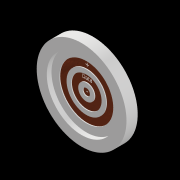
# Autodesk Inventor part: Connector
Saved by Autodesk Inventor 2022.1 (Build 261234000, 234)
## iProperties
Created: 2022-01-31
Part Number: Connector
Material: Generic
Document SubType Name: Modeling
Designer: Michael Lacey
Mass: 1.54155 g
Surface Area: 15.3616 cm^2
Volume: 1.54155 cm^3
Density: 1 g/cm^3
Appearance: Default
Author: Michael Lacey
Autodesk Inventor part; units mm, degrees
ref_plane "YZ Plane" through (0, 0, 0) normal (1, 0, 0) x (0, 1, 0)
ref_plane "XZ Plane" through (0, 0, 0) normal (0, 1, 0) x (-1, 0, 0)
ref_plane "XY Plane" through (0, 0, 0) normal (0, 0, 1) x (1, 0, 0)
sketch "Sketch1" plane through (0, 0, 0) normal (0, 0, 1) x (1, 0, 0)
  circle A0 centre (0, 0) radius 12.7 projected
  circle A1 centre (0, 0) radius 11.1125 construction
  circle A2 centre (0, 0) radius 9.8425
  dimension "d0" = 1.27
  constraints: 1 centre point, 1 coincident
  measures "d0" radial gap between concentric circles of A1 A2
extrude "Extrusion1" add sketch "Sketch1" along normal blind 3.175
sketch "Sketch2" plane through (0, 0, 0) normal (0, 0, -1) x (-1, 0, 0)
  circle A0 centre (0, 0) radius 1.016
  circle A1 centre (0, 0) radius 2.286
  circle A2 centre (0, 0) radius 4.318
  circle A3 centre (0, 0) radius 5.588
  circle A4 centre (0, 0) radius 7.62
  dimension "d3" = 2.032
  dimension "d4" = 2.032
  dimension "d5" = 2.032
  dimension "d6" = 1.27
  dimension "d7" = 1.27
  constraints: 5 centre point, 5 coincident
  measures "d3" diameter of A0
  measures "d4" radial gap between concentric circles of A2 A1
  measures "d5" radial gap between concentric circles of A4 A3
  measures "d6" radial gap between concentric circles of A1 A0
  measures "d7" radial gap between concentric circles of A3 A2
extrude "Extrusion2" add sketch "Sketch2" along normal mid plane 3.175
sketch "Sketch3" plane through (0, 0, 1.5875) normal (0, 0, 1) x (1, 0, 0)
  line L0 (-0.635, 7.239) -> (0.635, 7.239) construction
  line L1 (0.635, 7.239) -> (0.635, 5.969) construction
  line L2 (0.635, 5.969) -> (-0.635, 5.969) construction
  line L3 (-0.635, 5.969) -> (-0.635, 7.239) construction
  circle A0 centre (0, 0) radius 7.62 projected
  circle A1 centre (0, 0) radius 5.588 projected
  circle A2 centre (0, 0) radius 4.318 projected
  circle A3 centre (0, 0) radius 2.286 projected
  circle A4 centre (0, 0) radius 1.016 projected
  line L4 (0, 5.588) -> (0, 5.969) construction
  line L5 (0, 7.239) -> (0, 7.62) construction
  line L6 (-0.2762, 0.2762) -> (0.2762, 0.2762) construction
  line L7 (0.2762, 0.2762) -> (0.2762, -0.2762) construction
  line L8 (0.2762, -0.2762) -> (-0.2762, -0.2762) construction
  line L9 (-0.2762, -0.2762) -> (-0.2762, 0.2762) construction
  line L10 (0, 0.2762) -> (0, 1.016) construction
  line L11 (0.2762, 0) -> (1.016, 0) construction
  line L12 (0, -0.2762) -> (0, -1.016) construction
  line L13 (-0.2762, 0) -> (-1.016, 0) construction
  line L14 (-1.016, 4.318) -> (1.016, 4.318) construction
  line L15 (1.016, 4.318) -> (1.016, 2.286) construction
  line L16 (1.016, 2.286) -> (-1.016, 2.286) construction
  line L17 (-1.016, 2.286) -> (-1.016, 4.318) construction
  line L18 (0.5017, 6.5356) -> (0.0715, 6.5356)
  line L19 (0.0715, 6.5356) -> (0.0715, 6.1054)
  line L20 (0.0715, 6.1054) -> (-0.0705, 6.1054)
  line L21 (-0.0705, 6.1054) -> (-0.0705, 6.5356)
  line L22 (-0.0705, 6.5356) -> (-0.5007, 6.5356)
  line L23 (-0.5007, 6.5356) -> (-0.5007, 6.6724)
  line L24 (-0.5007, 6.6724) -> (-0.0705, 6.6724)
  line L25 (-0.0705, 6.6724) -> (-0.0705, 7.1026)
  line L26 (-0.0705, 7.1026) -> (0.0715, 7.1026)
  line L27 (0.0715, 7.1026) -> (0.0715, 6.6724)
  line L28 (0.0715, 6.6724) -> (0.5017, 6.6724)
  line L29 (0.5017, 6.6724) -> (0.5017, 6.5356)
  spline S0 degree 2 poles (-0.5372, 3.3119) (-0.5372, 3.1727) (-0.65, 2.9488) (-0.7447, 2.8862) knots 0 0 0 1 2 2 2
  spline S1 degree 2 poles (-0.7447, 2.8862) (-0.8221, 2.8376) (-0.981, 2.8047) (-1.1045, 2.8047) knots 0 0 0 1 2 2 2
  line L30 (-1.1045, 2.8047) -> (-1.3383, 2.8047)
  line L31 (-1.3383, 2.8047) -> (-1.3383, 3.8207)
  line L32 (-1.3383, 3.8207) -> (-1.107, 3.8207)
  spline S2 degree 2 poles (-1.107, 3.8207) (-0.9637, 3.8207) (-0.8007, 3.7779) (-0.7431, 3.74) knots 0 0 0 1 2 2 2
  spline S3 degree 2 poles (-0.7431, 3.74) (-0.6451, 3.675) (-0.5372, 3.4601) (-0.5372, 3.3119) knots 0 0 0 1 2 2 2
  spline S4 degree 2 poles (-0.678, 3.3135) (-0.678, 3.4304) (-0.7554, 3.5959) (-0.832, 3.6429) knots 0 0 0 1 2 2 2
  spline S5 degree 2 poles (-0.832, 3.6429) (-0.8863, 3.675) (-1.009, 3.7038) (-1.1004, 3.7038) knots 0 0 0 1 2 2 2
  line L33 (-1.1004, 3.7038) -> (-1.2033, 3.7038)
  line L34 (-1.2033, 3.7038) -> (-1.2033, 2.9216)
  line L35 (-1.2033, 2.9216) -> (-1.1004, 2.9216)
  spline S6 degree 2 poles (-1.1004, 2.9216) (-1.0106, 2.9216) (-0.8748, 2.9504) (-0.8196, 2.9891) knots 0 0 0 1 2 2 2
  spline S7 degree 2 poles (-0.8196, 2.9891) (-0.7488, 3.0369) (-0.678, 3.195) (-0.678, 3.3135) knots 0 0 0 1 2 2 2
  spline S8 degree 2 poles (0.0243, 2.8854) (0.0086, 2.8739) (-0.044, 2.8327) (-0.0687, 2.8203) knots 0 0 0 1 2 2 2
  spline S9 degree 2 poles (-0.0687, 2.8203) (-0.1025, 2.8022) (-0.1659, 2.7833) (-0.2235, 2.7833) knots 0 0 0 1 2 2 2
  spline S10 degree 2 poles (-0.2235, 2.7833) (-0.2705, 2.7833) (-0.3553, 2.8187) (-0.3874, 2.8508) knots 0 0 0 1 2 2 2
  spline S11 degree 2 poles (-0.3874, 2.8508) (-0.4178, 2.8821) (-0.4549, 2.9743) (-0.4549, 3.0254) knots 0 0 0 1 2 2 2
  spline S12 degree 2 poles (-0.4549, 3.0254) (-0.4549, 3.1044) (-0.3882, 3.2164) (-0.3158, 3.2485) knots 0 0 0 1 2 2 2
  spline S13 degree 2 poles (-0.3158, 3.2485) (-0.2515, 3.2781) (-0.077, 3.3004) (0.0243, 3.3061) knots 0 0 0 1 2 2 2
  line L36 (0.0243, 3.3061) -> (0.0243, 3.3308)
  spline S14 degree 2 poles (0.0243, 3.3308) (0.0243, 3.3753) (-0.0029, 3.4304) (-0.0276, 3.4461) knots 0 0 0 1 2 2 2
  spline S15 degree 2 poles (-0.0276, 3.4461) (-0.0523, 3.4617) (-0.1231, 3.4716) (-0.161, 3.4716) knots 0 0 0 1 2 2 2
  spline S16 degree 2 poles (-0.161, 3.4716) (-0.2054, 3.4716) (-0.3256, 3.4453) (-0.3857, 3.4197) knots 0 0 0 1 2 2 2
  line L37 (-0.3857, 3.4197) -> (-0.3931, 3.4197)
  line L38 (-0.3931, 3.4197) -> (-0.3931, 3.5506)
  spline S17 degree 2 poles (-0.3931, 3.5506) (-0.3577, 3.5605) (-0.2252, 3.5852) (-0.1601, 3.5852) knots 0 0 0 1 2 2 2
  spline S18 degree 2 poles (-0.1601, 3.5852) (-0.0811, 3.5852) (0.0268, 3.5605) (0.0696, 3.5284) knots 0 0 0 1 2 2 2
  spline S19 degree 2 poles (0.0696, 3.5284) (0.1116, 3.4971) (0.1527, 3.3975) (0.1527, 3.3259) knots 0 0 0 1 2 2 2
  line L39 (0.1527, 3.3259) -> (0.1527, 2.8047)
  line L40 (0.1527, 2.8047) -> (0.0243, 2.8047)
  line L41 (0.0243, 2.8047) -> (0.0243, 2.8854)
  line L42 (0.0243, 2.9924) -> (0.0243, 3.204)
  spline S20 degree 2 poles (0.0243, 3.204) (-0.0218, 3.1999) (-0.161, 3.1859) (-0.2046, 3.1727) knots 0 0 0 1 2 2 2
  spline S21 degree 2 poles (-0.2046, 3.1727) (-0.2556, 3.1571) (-0.3223, 3.092) (-0.3223, 3.0344) knots 0 0 0 1 2 2 2
  spline S22 degree 2 poles (-0.3223, 3.0344) (-0.3223, 2.9685) (-0.2482, 2.9019) (-0.1774, 2.9019) knots 0 0 0 1 2 2 2
  spline S23 degree 2 poles (-0.1774, 2.9019) (-0.1173, 2.9019) (-0.0185, 2.9537) (0.0243, 2.9924) knots 0 0 0 1 2 2 2
  spline S24 degree 2 poles (0.5636, 2.7899) (0.459, 2.7899) (0.3413, 2.9093) (0.3413, 3.0385) knots 0 0 0 1 2 2 2
  line L43 (0.3413, 3.0385) -> (0.3413, 3.4609)
  line L44 (0.3413, 3.4609) -> (0.2548, 3.4609)
  line L45 (0.2548, 3.4609) -> (0.2548, 3.5671)
  line L46 (0.2548, 3.5671) -> (0.3413, 3.5671)
  line L47 (0.3413, 3.5671) -> (0.3413, 3.7861)
  line L48 (0.3413, 3.7861) -> (0.4697, 3.7861)
  line L49 (0.4697, 3.7861) -> (0.4697, 3.5671)
  line L50 (0.4697, 3.5671) -> (0.706, 3.5671)
  line L51 (0.706, 3.5671) -> (0.706, 3.4609)
  line L52 (0.706, 3.4609) -> (0.4697, 3.4609)
  line L53 (0.4697, 3.4609) -> (0.4697, 3.0978)
  spline S25 degree 2 poles (0.4697, 3.0978) (0.4697, 3.0402) (0.4738, 2.9768) (0.4878, 2.9496) knots 0 0 0 1 2 2 2
  spline S26 degree 2 poles (0.4878, 2.9496) (0.4994, 2.9257) (0.5512, 2.9019) (0.5957, 2.9019) knots 0 0 0 1 2 2 2
  spline S27 degree 2 poles (0.5957, 2.9019) (0.627, 2.9019) (0.6854, 2.9208) (0.6986, 2.9266) knots 0 0 0 1 2 2 2
  line L54 (0.6986, 2.9266) -> (0.706, 2.9266)
  line L55 (0.706, 2.9266) -> (0.706, 2.8113)
  spline S28 degree 2 poles (0.706, 2.8113) (0.6698, 2.8014) (0.5957, 2.7899) (0.5636, 2.7899) knots 0 0 0 1 2 2 2
  spline S29 degree 2 poles (1.2255, 2.8854) (1.2099, 2.8739) (1.1572, 2.8327) (1.1325, 2.8203) knots 0 0 0 1 2 2 2
  spline S30 degree 2 poles (1.1325, 2.8203) (1.0987, 2.8022) (1.0353, 2.7833) (0.9777, 2.7833) knots 0 0 0 1 2 2 2
  spline S31 degree 2 poles (0.9777, 2.7833) (0.9308, 2.7833) (0.846, 2.8187) (0.8139, 2.8508) knots 0 0 0 1 2 2 2
  spline S32 degree 2 poles (0.8139, 2.8508) (0.7834, 2.8821) (0.7464, 2.9743) (0.7464, 3.0254) knots 0 0 0 1 2 2 2
  spline S33 degree 2 poles (0.7464, 3.0254) (0.7464, 3.1044) (0.813, 3.2164) (0.8855, 3.2485) knots 0 0 0 1 2 2 2
  spline S34 degree 2 poles (0.8855, 3.2485) (0.9497, 3.2781) (1.1243, 3.3004) (1.2255, 3.3061) knots 0 0 0 1 2 2 2
  line L56 (1.2255, 3.3061) -> (1.2255, 3.3308)
  spline S35 degree 2 poles (1.2255, 3.3308) (1.2255, 3.3753) (1.1984, 3.4304) (1.1737, 3.4461) knots 0 0 0 1 2 2 2
  spline S36 degree 2 poles (1.1737, 3.4461) (1.149, 3.4617) (1.0782, 3.4716) (1.0403, 3.4716) knots 0 0 0 1 2 2 2
  spline S37 degree 2 poles (1.0403, 3.4716) (0.9958, 3.4716) (0.8756, 3.4453) (0.8155, 3.4197) knots 0 0 0 1 2 2 2
  line L57 (0.8155, 3.4197) -> (0.8081, 3.4197)
  line L58 (0.8081, 3.4197) -> (0.8081, 3.5506)
  spline S38 degree 2 poles (0.8081, 3.5506) (0.8435, 3.5605) (0.9761, 3.5852) (1.0411, 3.5852) knots 0 0 0 1 2 2 2
  spline S39 degree 2 poles (1.0411, 3.5852) (1.1202, 3.5852) (1.228, 3.5605) (1.2708, 3.5284) knots 0 0 0 1 2 2 2
  spline S40 degree 2 poles (1.2708, 3.5284) (1.3128, 3.4971) (1.354, 3.3975) (1.354, 3.3259) knots 0 0 0 1 2 2 2
  line L59 (1.354, 3.3259) -> (1.354, 2.8047)
  line L60 (1.354, 2.8047) -> (1.2255, 2.8047)
  line L61 (1.2255, 2.8047) -> (1.2255, 2.8854)
  line L62 (1.2255, 2.9924) -> (1.2255, 3.204)
  spline S41 degree 2 poles (1.2255, 3.204) (1.1794, 3.1999) (1.0403, 3.1859) (0.9967, 3.1727) knots 0 0 0 1 2 2 2
  spline S42 degree 2 poles (0.9967, 3.1727) (0.9456, 3.1571) (0.8789, 3.092) (0.8789, 3.0344) knots 0 0 0 1 2 2 2
  spline S43 degree 2 poles (0.8789, 3.0344) (0.8789, 2.9685) (0.953, 2.9019) (1.0238, 2.9019) knots 0 0 0 1 2 2 2
  spline S44 degree 2 poles (1.0238, 2.9019) (1.0839, 2.9019) (1.1827, 2.9537) (1.2255, 2.9924) knots 0 0 0 1 2 2 2
  line L63 (0.2408, -0.0772) -> (-0.2398, -0.0772)
  line L64 (-0.2398, -0.0772) -> (-0.2398, 0.0772)
  line L65 (-0.2398, 0.0772) -> (0.2408, 0.0772)
  line L66 (0.2408, 0.0772) -> (0.2408, -0.0772)
  point P0 (0, 2.286)
  point P1 (0, 4.318)
  point P2 (2.886, -2.4456)
  point P3 (2.886, 0.3842)
  dimension "d12" = 1.27
  constraints: 12 end point, 8 midpoint, 6 equal length, 6 vertical alignment, 4 point on circle, 3 horizontal, 2 point on line, 2 vertical, 1 horizontal alignment, 10 other
  measures "d12" distance of L0.end L1.end
extrude "Extrusion3" cut sketch "Sketch3" against normal blind 0.508 contours L18 L19 L20 L21 L22 L23 L24 L25 L26 L27 L28 L29 | S0 S1 L30 L31 L32 S2 S3 | S8 S9 S10 S11 S12 S13 L36 S14 S15 S16 L37 L38 S17 S18 S19 L39 L40 L41 | S24 L43 L44 L45 L46 L47 L48 L49 L50 L51 L52 L53 S25 S26 S27 L54 L55 S28 | S29 S30 S31 S32 S33 S34 L56 S35 S36 S37 L57 L58 S38 S39 S40 L59 L60 L61 | L63 L64 L65 L66
sketch "Sketch4" plane through (0, 0, 1.5875) normal (0, 0, 1) x (1, 0, 0)
  circle A0 centre (0, 0) radius 2.286 projected
  circle A1 centre (0, 0) radius 4.318 projected
  line L0 (1.2255, 2.8047) -> (1.2255, 2.8854) projected
  line L1 (1.2255, 3.3061) -> (1.2255, 3.3308) projected
  line L2 (0.8155, 3.4197) -> (0.8081, 3.4197) projected
  line L3 (0.8081, 3.4197) -> (0.8081, 3.5506) projected
  line L4 (1.354, 3.3259) -> (1.354, 2.8047) projected
  line L5 (1.354, 2.8047) -> (1.2255, 2.8047) projected
  line L6 (-1.1045, 2.8047) -> (-1.3383, 2.8047) projected
  line L7 (-1.3383, 2.8047) -> (-1.3383, 3.8207) projected
  line L8 (-1.3383, 3.8207) -> (-1.107, 3.8207) projected
  line L9 (0.0243, 2.8047) -> (0.0243, 2.8854) projected
  line L10 (0.0243, 3.3061) -> (0.0243, 3.3308) projected
  line L11 (-0.3857, 3.4197) -> (-0.3931, 3.4197) projected
  line L12 (-0.3931, 3.4197) -> (-0.3931, 3.5506) projected
  line L13 (0.1527, 3.3259) -> (0.1527, 2.8047) projected
  line L14 (0.1527, 2.8047) -> (0.0243, 2.8047) projected
  line L15 (0.3413, 3.0385) -> (0.3413, 3.4609) projected
  line L16 (0.3413, 3.4609) -> (0.2548, 3.4609) projected
  line L17 (0.2548, 3.4609) -> (0.2548, 3.5671) projected
  line L18 (0.2548, 3.5671) -> (0.3413, 3.5671) projected
  line L19 (0.3413, 3.5671) -> (0.3413, 3.7861) projected
  line L20 (0.3413, 3.7861) -> (0.4697, 3.7861) projected
  line L21 (0.4697, 3.7861) -> (0.4697, 3.5671) projected
  line L22 (0.4697, 3.5671) -> (0.706, 3.5671) projected
  line L23 (0.706, 3.5671) -> (0.706, 3.4609) projected
  line L24 (0.706, 3.4609) -> (0.4697, 3.4609) projected
  line L25 (0.4697, 3.4609) -> (0.4697, 3.0978) projected
  line L26 (0.6986, 2.9266) -> (0.706, 2.9266) projected
  line L27 (0.706, 2.9266) -> (0.706, 2.8113) projected
  line L28 (0.5017, 6.6724) -> (0.5017, 6.5356) projected
  line L29 (0.5017, 6.5356) -> (0.0715, 6.5356) projected
  line L30 (0.0715, 6.5356) -> (0.0715, 6.1054) projected
  line L31 (0.0715, 6.1054) -> (-0.0705, 6.1054) projected
  line L32 (-0.0705, 6.1054) -> (-0.0705, 6.5356) projected
  line L33 (-0.0705, 6.5356) -> (-0.5007, 6.5356) projected
  line L34 (-0.5007, 6.5356) -> (-0.5007, 6.6724) projected
  line L35 (-0.5007, 6.6724) -> (-0.0705, 6.6724) projected
  line L36 (-0.0705, 6.6724) -> (-0.0705, 7.1026) projected
  line L37 (-0.0705, 7.1026) -> (0.0715, 7.1026) projected
  line L38 (0.0715, 7.1026) -> (0.0715, 6.6724) projected
  line L39 (0.0715, 6.6724) -> (0.5017, 6.6724) projected
  circle A2 centre (0, 0) radius 7.62 projected
  circle A3 centre (0, 0) radius 5.588 projected
  line L40 (0.2408, 0.0772) -> (0.2408, -0.0772) projected
  line L41 (0.2408, -0.0772) -> (-0.2398, -0.0772) projected
  line L42 (-0.2398, -0.0772) -> (-0.2398, 0.0772) projected
  line L43 (-0.2398, 0.0772) -> (0.2408, 0.0772) projected
  circle A4 centre (0, 0) radius 1.016 projected
  circle A5 centre (0, 0) radius 12.7 projected
  circle A6 centre (0, 0) radius 9.8425 projected
  point P0 (1.1325, 2.8203)
  point P1 (0.9777, 2.7833)
  point P2 (0.8139, 2.8508)
  point P3 (0.7464, 3.0254)
  point P4 (0.8855, 3.2485)
  point P5 (1.1737, 3.4461)
  point P6 (1.0403, 3.4716)
  point P7 (1.0411, 3.5852)
  point P8 (1.2708, 3.5284)
  point P9 (-0.7431, 3.74)
  point P10 (-0.5372, 3.3119)
  point P11 (-0.7447, 2.8862)
  point P12 (-0.0687, 2.8203)
  point P13 (-0.2235, 2.7833)
  point P14 (-0.3874, 2.8508)
  point P15 (-0.4549, 3.0254)
  point P16 (-0.3158, 3.2485)
  point P17 (-0.0276, 3.4461)
  point P18 (-0.161, 3.4716)
  point P19 (-0.1601, 3.5852)
  point P20 (0.0696, 3.5284)
  point P21 (0.5636, 2.7899)
  point P22 (0.4878, 2.9496)
  point P23 (0.5957, 2.9019)
  constraints: 33 other
extrude "Extrusion4" add sketch "Sketch4" along normal blind 0.254 and the other way blind 2.54 contours A0 | A3 | A6
body "Solid1"
